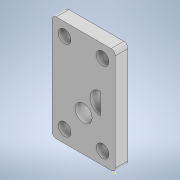
# Autodesk Inventor part: zad 7
Saved by Autodesk Inventor 2020 (Build 240168000, 168)
## iProperties
Created: 2022-03-14
Part Number: zad 7
Material: Ogólny
Document SubType Name: Modeling
Designer: 3IG
Density: 1 g/cm^3
Appearance: Domyślna
Author: 3IG
Autodesk Inventor part; units mm, degrees
ref_plane "YZ Plane" through (0, 0, 0) normal (1, 0, 0) x (0, 1, 0)
ref_plane "XZ Plane" through (0, 0, 0) normal (0, 1, 0) x (-1, 0, 0)
ref_plane "XY Plane" through (0, 0, 0) normal (0, 0, 1) x (1, 0, 0)
sketch "Szkic1" plane through (0, 0, 0) normal (0, 0, 1) x (1, 0, 0)
  line L0 (-1, 0) -> (-14, 0)
  line L1 (-15, 1) -> (-15, 24)
  line L2 (-14, 25) -> (-1, 25)
  line L3 (0, 24) -> (0, 1)
  arc A0 (-14, 25) -> (-15, 24) centre (-14, 24) ccw
  arc A1 (0, 24) -> (-1, 25) centre (-1, 24) ccw
  arc A2 (-1, 0) -> (0, 1) centre (-1, 1) ccw
  arc A3 (-15, 1) -> (-14, 0) centre (-14, 1) ccw
  circle A4 centre (-3, 3) radius 1.5
  circle A5 centre (-12, 3) radius 1.5
  circle A6 centre (-12, 22) radius 1.5
  circle A7 centre (-3, 22) radius 1.5
  line L4 (-3.5, 15) -> (-3.5, 10)
  circle A8 centre (-7.5, 8.5) radius 2
  arc A9 (-3.5, 15) -> (-3.5, 10) centre (-3.5, 12.5) ccw
  point P0 (0, 0)
  point P1 (-15, 25)
  point P2 (-15, 0)
  point P3 (0, 25)
  point P4 (-11.5, 20.5)
  point P5 (-11.5, 4.5)
  point P6 (-3.5, 20.5)
  dimension "d0" = 15
  dimension "d1" = 25
  dimension "d2" = 1
  dimension "d3" = 3
  dimension "d4" = 3
  dimension "d5" = 3
  dimension "d6" = 3
  dimension "d7" = 8
  dimension "d8" = 16
  dimension "d10" = 19
  dimension "d11" = 4
  constraints: 10 centre point, 10 end point, 10 point on circle, 9 point on line, 8 tangent, 3 equal radius, 2 parallel, 1 horizontal, 1 midpoint, 1 perpendicular
  measures "d0" distance of point (-15, 25) point (0, 25)
  measures "d1" distance of point (-15, 0) point (-15, 25)
  measures "d2" radius of A0
  measures "d3" diameter of A4
  measures "d4" diameter of A5
  measures "d5" diameter of A6
  measures "d6" diameter of A7
  measures "d7" distance of point (-11.5, 20.5) point (-3.5, 20.5)
  measures "d8" distance of point (-11.5, 4.5) point (-11.5, 20.5)
  measures "d10" distance of A4.centre A7.centre
  measures "d11" diameter of A8
extrude "Wyciągnięcie proste1" add sketch "Szkic1" along normal blind 3
sketch "Szkic2" plane through (0, 0, 3) normal (0, 0, 1) x (1, 0, 0)
  point P0 (0, 0)
sketch "Szkic3" plane through (0, 0, 3) normal (0, 0, 1) x (1, 0, 0)
  point P0 (0, 0)
sketch "Szkic4" plane through (0, 0, 3) normal (0, 0, 1) x (1, 0, 0)
  point P0 (0, 0)
